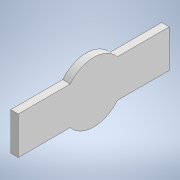
# Autodesk Inventor part: leg_base_plate
Saved by Autodesk Inventor 2022.5 (Build 265521000, 521)
## iProperties
Created: 2024-06-27
Part Number: leg_base_plate
Material: 一般
Document SubType Name: Modeling
Designer: gakut
Density: 1 g/cm^3
Appearance: 既定
Author: gakut
Autodesk Inventor part; units mm, degrees
ref_plane "YZ Plane" through (0, 0, 0) normal (1, 0, 0) x (0, 1, 0)
ref_plane "XZ Plane" through (0, 0, 0) normal (0, 1, 0) x (-1, 0, 0)
ref_plane "XY Plane" through (0, 0, 0) normal (0, 0, 1) x (1, 0, 0)
sketch "スケッチ1" plane through (0, 0, 0) normal (1, 0, 0) x (0, 1, 0)
  circle A0 centre (0, 0) radius 40
  line L0 (-25, 100) -> (25, 100)
  line L1 (25, 100) -> (25, -100)
  line L2 (25, -100) -> (-25, -100)
  line L3 (-25, -100) -> (-25, 100)
  line L4 (-25, 100) -> (25, -100) construction
  line L5 (25, 100) -> (-25, -100) construction
  point P0 (25, -31.225)
  point P1 (25, 31.225)
  point P2 (-25, 31.225)
  point P3 (-25, -31.225)
  dimension "d0" = 80
  dimension "d1" = 50
  dimension "d2" = 200
  constraints: 12 end point, 2 midpoint, 2 parallel, 1 centre point, 1 coincident, 1 horizontal, 1 perpendicular
  measures "d0" diameter of A0
  measures "d1" distance of L1.end L2.end
  measures "d2" distance of L0.end L1.end
extrude "押し出し1" add sketch "スケッチ1" along normal blind 10
ref_plane "作業平面1" through (0, -25, 0) normal (0, 0, 1) x (1, 0, 0)
